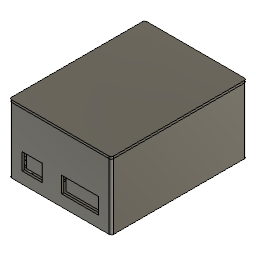
Case (Autodesk Fusion 360 design; units mm, degrees)
Autodesk Fusion 360 part; units mm, degrees
sketch "Base" plane through (0, 0, 0) normal (0, 0, 1) x (1, 0, 0) in component "PCB"
  line L0 (58.9, 60.9) -> (0, 60.9)
  line L1 (0, 60.9) -> (0, 0)
  line L2 (0, 0) -> (58.9, 0)
  line L3 (58.9, 0) -> (58.9, 60.9)
  circle A0 centre (3.45, 57.45) radius 1.6
  line L4 (29.45, 60.9) -> (29.45, 0) construction
  line L5 (0, 30.45) -> (58.9, 30.45) construction
  circle A1 centre (55.45, 57.45) radius 1.6
  circle A2 centre (3.45, 3.45) radius 1.6
  circle A3 centre (55.45, 3.45) radius 1.6
  dimension "d1" = 58.9
  dimension "d2" = 60.9
  dimension "d3" = 3.2
  dimension "d4" = 3.45
  dimension "d5" = 3.45
  constraint horizontal L0
  constraint vertical L1
  constraint horizontal L2
  constraint vertical L3
  constraint coincident L1.end L2.start
  constraint midpoint L0 L4.start
  constraint midpoint L2 L4.end
  constraint midpoint L1 L5.start
  constraint midpoint L3 L5.end
  constraint symmetric A0 L4 A1
  constraint symmetric A0 L5 A2
  constraint symmetric L5 A1 A3
  measures "d1" distance of L1.end L2.end
  measures "d2" distance of L0.end L1.end
  measures "d3" diameter of A0
  measures "d4" distance of L0 A0.centre
  measures "d5" distance of L1 A0.centre
extrude "Extrude1" add sketch "Base" along normal blind 24.2 makes body 1 in component "PCB"
sketch "USB port" plane through (0, 60.9, 0) normal (0, 1, 0) x (-1, 0, 0) in component "PCB"
  line L0 (-58.9, 0) -> (0, 0)
  line L1 (0, 0) -> (0, 24.2)
  line L2 (0, 24.2) -> (-58.9, 24.2)
  line L3 (-58.9, 24.2) -> (-58.9, 0)
  line L4 (-44.9, 16.5) -> (-36.9, 16.5)
  line L5 (-36.9, 16.5) -> (-36.9, 13.5)
  line L6 (-36.9, 13.5) -> (-44.9, 13.5)
  line L7 (-44.9, 13.5) -> (-44.9, 16.5)
  dimension "d8" = 8
  dimension "d9" = 3
  dimension "d10" = 14
  dimension "d11" = 13.5
  constraint horizontal L4
  constraint vertical L5
  constraint horizontal L6
  constraint vertical L7
  measures "d8" distance of L4.start L4.end
  measures "d9" distance of L4.start L6.end
  measures "d10" distance of L3 L7
  measures "d11" distance of L0 L6
extrude "Extrude2" add sketch "USB port" along normal blind 1 contours L4 L5 L6 L7 bodies 1 in component "PCB"
sketch "Base (2)" plane through (0, 0, 0) normal (0, 0, 1) x (1, 0, 0) in component "RJ45 breakout"
  line L0 (35.9, 21.4) -> (0, 21.4)
  line L1 (0, 21.4) -> (0, 0)
  line L2 (0, 0) -> (35.9, 0)
  line L3 (35.9, 0) -> (35.9, 21.4)
  circle A0 centre (4, 5) radius 1.6
  line L4 (17.95, 21.4) -> (17.95, 0) construction
  circle A1 centre (31.9, 5) radius 1.6
  dimension "d14" = 35.9
  dimension "d15" = 21.4
  dimension "d16" = 3.2
  dimension "d17" = 5
  dimension "d18" = 4
  constraint horizontal L0
  constraint vertical L1
  constraint horizontal L2
  constraint vertical L3
  constraint coincident L1.end L2.start
  constraint midpoint L0 L4.start
  constraint midpoint L2 L4.end
  constraint symmetric A0 L4 A1
  measures "d14" distance of L0.start L0.end
  measures "d15" distance of L0.end L1.end
  measures "d16" diameter of A0
  measures "d17" distance of L2 A0.centre
  measures "d18" distance of L1 A0.centre
extrude "Extrude1'" add sketch "Base (2)" along normal blind 1.5 separate body makes body 2 in component "RJ45 breakout"
sketch "Port" plane through (0, 0, 1.5) normal (0, 0, 1) x (-1, 0, 0) in component "RJ45 breakout"
  circle A0 centre (-31.9, -5) radius 1.6
  circle A1 centre (-4, -5) radius 1.6
  line L0 (-35.9, 0) -> (-35.9, -21.4)
  line L1 (-35.9, -21.4) -> (0, -21.4)
  line L2 (0, -21.4) -> (0, 0)
  line L3 (0, 0) -> (-35.9, 0)
  line L4 (-9.8, -13.3) -> (-26.1, -13.3)
  line L5 (-26.1, -13.3) -> (-26.1, 2.1)
  line L6 (-26.1, 2.1) -> (-9.8, 2.1)
  line L7 (-9.8, 2.1) -> (-9.8, -13.3)
  dimension "d21" = 16.3
  dimension "d22" = 15.4
  dimension "d23" = 2.1
  dimension "d24" = 35.9
  dimension "d25" = 9.8
  constraint horizontal L4
  constraint vertical L5
  constraint horizontal L6
  constraint vertical L7
  measures "d21" distance of L4.start L4.end
  measures "d22" distance of L4.start L6.end
  measures "d23" distance of L3 L6
  measures "d24" distance of L0.end L1.end
  measures "d25" distance of L2 L7
extrude "Extrude2'" add sketch "Port" along normal blind 13.3 contours L3 L5 L6 L7 | L3 L4 L5 L7 bodies 2 in component "RJ45 breakout"
sketch "Base (3)" plane through (0, 0, 0) normal (0, 0, 1) x (1, 0, 0) in component "UART to RS-232 converter"
  line L0 (31.6, 28) -> (0, 28)
  line L1 (0, 28) -> (0, 0)
  line L2 (0, 0) -> (31.6, 0)
  line L3 (31.6, 0) -> (31.6, 28)
  circle A0 centre (2.1, 25.7) radius 1.6
  line L4 (15.8, 28) -> (15.8, 0) construction
  circle A1 centre (29.5, 25.7) radius 1.6
  dimension "d28" = 28
  dimension "d29" = 31.6
  dimension "d30" = 3.2
  dimension "d31" = 2.1
  dimension "d32" = 2.3
  constraint horizontal L0
  constraint vertical L1
  constraint horizontal L2
  constraint vertical L3
  constraint coincident L1.end L2.start
  constraint midpoint L0 L4.start
  constraint midpoint L2 L4.end
  constraint symmetric A0 L4 A1
  measures "d28" distance of L0.end L1.end
  measures "d29" distance of L0.start L0.end
  measures "d30" diameter of A0
  measures "d31" distance of L1 A0.centre
  measures "d32" distance of L0 A0.centre
extrude "Extrude1''" add sketch "Base (3)" along normal blind 1.5 separate body makes body 3 in component "UART to RS-232 converter"
sketch "Port (2)" plane through (0, 0, 1.5) normal (0, 0, 1) x (-1, 0, 0) in component "UART to RS-232 converter"
  circle A0 centre (-29.5, -25.7) radius 1.6
  circle A1 centre (-2.1, -25.7) radius 1.6
  line L0 (-31.6, 0) -> (-31.6, -28)
  line L1 (-31.6, -28) -> (0, -28)
  line L2 (0, -28) -> (0, 0)
  line L3 (0, 0) -> (-31.6, 0)
  line L4 (0, -12.3) -> (-31.6, -12.3)
  line L5 (-31.6, -12.3) -> (-31.6, 17.9)
  line L6 (-31.6, 17.9) -> (0, 17.9)
  line L7 (0, 17.9) -> (0, -12.3)
  dimension "d35" = 30.2
  dimension "d36" = 12.3
  constraint horizontal L4
  constraint vertical L5
  constraint horizontal L6
  constraint vertical L7
  constraint collinear L2 L7
  constraint collinear L0 L5
  measures "d35" distance of L4.start L6.end
  measures "d36" distance of L3 L4
extrude "Extrude2''" add sketch "Port (2)" along normal blind 12.7 contours L0 L2 L3 L4 L5 L7 | L3 L5 L6 L7 bodies 3 in component "UART to RS-232 converter"
other "GeometricRelationship6"
sketch "Base (4)" plane through (0, 0, 0) normal (0, 0, 1) x (1, 0, 0) in component "Case"
  line L0 (-24.1768, 62.9) -> (65.1232, 62.9)
  line L1 (65.1232, 62.9) -> (65.1232, -56.9)
  line L2 (65.1232, -56.9) -> (-24.1768, -56.9)
  line L3 (-24.1768, -56.9) -> (-24.1768, 62.9)
  line L4 (-26.1768, 64.9) -> (67.1232, 64.9)
  line L5 (67.1232, 64.9) -> (67.1232, -58.9)
  line L6 (67.1232, -58.9) -> (-26.1768, -58.9)
  line L7 (-26.1768, -58.9) -> (-26.1768, 64.9)
  point P0 (-23.1768, -53.8)
  point P1 (54.3232, -55.9)
  point P2 (44.9, 61.9)
  point P3 (-13.3768, -55.9)
  dimension "d63" = 1
  dimension "d64" = 1
  dimension "d65" = 10.8
  dimension "d66" = 1
  dimension "d67" = 2
  dimension "d68" = 2
  dimension "d69" = 2
  dimension "d70" = 2
  dimension "d81" = 9.8
  constraint horizontal L0
  constraint vertical L1
  constraint horizontal L2
  constraint vertical L3
  constraint horizontal L4
  constraint vertical L5
  constraint horizontal L6
  constraint vertical L7
  measures "d63" distance of P0 L3
  measures "d64" distance of P1 L2
  measures "d65" distance of P1 L1
  measures "d66" distance of P2 L0
  measures "d67" distance of L0 L4
  measures "d68" distance of L3 L7
  measures "d69" distance of L1 L5
  measures "d70" distance of L2 L6
  measures "d81" horizontal distance of P0 P3
extrude "Extrude1'''" add sketch "Base (4)" along normal blind 10 separate body contours L0 L1 L2 L3 | L4 L5 L6 L7 makes body 4 in component "Case"
fillet "Fillet1" radius 2 4 edges at (67.1232, -58.9, 5) (67.1232, 64.9, 5) (-26.1768, 64.9, 5) (-26.1768, -58.9, 5) on bodies 4 in component "Case"
sketch "Walls" plane through (0, 0, 10) normal (0, 0, 1) x (-1, 0, 0) in component "Case"
  arc A0 (26.1768, 56.9) -> (24.1768, 58.9) centre (24.1768, 56.9) ccw
  line L0 (24.1768, 58.9) -> (-65.1232, 58.9)
  arc A1 (-65.1232, 58.9) -> (-67.1232, 56.9) centre (-65.1232, 56.9) ccw
  line L1 (-67.1232, 56.9) -> (-67.1232, -62.9)
  arc A2 (-67.1232, -62.9) -> (-65.1232, -64.9) centre (-65.1232, -62.9) ccw
  line L2 (-65.1232, -64.9) -> (24.1768, -64.9)
  arc A3 (24.1768, -64.9) -> (26.1768, -62.9) centre (24.1768, -62.9) ccw
  line L3 (26.1768, -62.9) -> (26.1768, 56.9)
  line L4 (24.1768, 56.9) -> (24.1768, -62.9)
  line L5 (-65.1232, 56.9) -> (24.1768, 56.9)
  line L6 (-65.1232, -62.9) -> (-65.1232, 56.9)
  line L7 (24.1768, -62.9) -> (-65.1232, -62.9)
extrude "Extrude2'''" add sketch "Walls" along normal blind 50 bodies 4 in component "Case"
other "GeometricRelationship8"
other "GeometricRelationship9"
sketch "Front port holes" plane through (0, -58.9, 0) normal (0, -1, 0) x (1, 0, 0) in component "Case"
  line L0 (-24.1768, 60) -> (-24.1768, 0)
  line L1 (-24.1768, 0) -> (65.1232, 0)
  line L2 (65.1232, 0) -> (65.1232, 60)
  line L3 (65.1232, 60) -> (-24.1768, 60)
  line L4 (-13.3768, 11.5) -> (2.9232, 11.5) construction
  line L5 (2.9232, 11.5) -> (2.9232, 24.8) construction
  line L6 (2.9232, 24.8) -> (-13.3768, 24.8) construction
  line L7 (-13.3768, 24.8) -> (-13.3768, 11.5) construction
  line L8 (22.7232, 11.5) -> (54.3232, 11.5) construction
  line L9 (54.3232, 11.5) -> (54.3232, 24.2) construction
  line L10 (54.3232, 24.2) -> (22.7232, 24.2) construction
  line L11 (22.7232, 24.2) -> (22.7232, 11.5) construction
  line L12 (-14.3768, 25.8) -> (3.9232, 25.8)
  line L13 (3.9232, 25.8) -> (3.9232, 10.5)
  line L14 (3.9232, 10.5) -> (-14.3768, 10.5)
  line L15 (-14.3768, 10.5) -> (-14.3768, 25.8)
  line L16 (21.7232, 25.2) -> (55.3232, 25.2)
  line L17 (55.3232, 25.2) -> (55.3232, 10.5)
  line L18 (55.3232, 10.5) -> (21.7232, 10.5)
  line L19 (21.7232, 10.5) -> (21.7232, 25.2)
  dimension "d82" = 1
  dimension "d83" = 1
  dimension "d84" = 1
  dimension "d85" = 1
  dimension "d86" = 1
  dimension "d87" = 1
  dimension "d88" = 1
  dimension "d89" = 1
  constraint horizontal L12
  constraint vertical L13
  constraint horizontal L14
  constraint vertical L15
  constraint horizontal L16
  constraint vertical L17
  constraint horizontal L18
  constraint vertical L19
  measures "d82" distance of L6 L12
  measures "d83" distance of L7 L15
  measures "d84" distance of L4 L14
  measures "d85" distance of L5 L13
  measures "d86" distance of L11 L19
  measures "d87" distance of L8 L18
  measures "d88" distance of L9 L17
  measures "d89" distance of L10 L16
extrude "Extrude3" cut sketch "Front port holes" against normal up to surface (2 mm away) contours L12 L13 L14 L15 | L16 L17 L18 L19 bodies 4 in component "Case"
sketch "Back port hole" plane through (0, 64.9, 0) normal (0, 1, 0) x (-1, 0, 0) in component "Case"
  line L0 (24.1768, 0) -> (24.1768, 60)
  line L1 (24.1768, 60) -> (-65.1232, 60)
  line L2 (-65.1232, 60) -> (-65.1232, 0)
  line L3 (-65.1232, 0) -> (24.1768, 0)
  line L4 (-35.9232, 23.5) -> (-27.9232, 23.5) construction
  line L5 (-27.9232, 23.5) -> (-27.9232, 26.5) construction
  line L6 (-27.9232, 26.5) -> (-35.9232, 26.5) construction
  line L7 (-35.9232, 26.5) -> (-35.9232, 23.5) construction
  line L8 (-37.9232, 29.5) -> (-25.9232, 29.5)
  line L9 (-25.9232, 29.5) -> (-25.9232, 20.5)
  line L10 (-25.9232, 20.5) -> (-37.9232, 20.5)
  line L11 (-37.9232, 20.5) -> (-37.9232, 29.5)
  dimension "d92" = 3
  dimension "d93" = 2
  dimension "d94" = 3
  dimension "d95" = 2
  constraint horizontal L8
  constraint vertical L9
  constraint horizontal L10
  constraint vertical L11
  measures "d92" distance of L6 L8
  measures "d93" distance of L7 L11
  measures "d94" distance of L4 L10
  measures "d95" distance of L5 L9
extrude "Extrude4" cut sketch "Back port hole" against normal up to surface (2 mm away) contours L8 L9 L10 L11 bodies 4 in component "Case"
sketch "Threaded insert holes" plane through (0, 0, 10) normal (0, 0, 1) x (-1, 0, 0) in component "Case"
  line L0 (24.1768, 56.9) -> (-65.1232, 56.9)
  line L1 (-65.1232, 56.9) -> (-65.1232, -62.9)
  line L2 (-65.1232, -62.9) -> (24.1768, -62.9)
  line L3 (24.1768, -62.9) -> (24.1768, 56.9)
  circle A0 centre (19.1768, 48.8) radius 1.6 construction
  circle A1 centre (-8.7232, 48.8) radius 1.6 construction
  circle A2 centre (-24.8232, 12.3) radius 1.6 construction
  circle A3 centre (-52.2232, 12.3) radius 1.6 construction
  circle A4 centre (-46.4732, -3.45) radius 1.6 construction
  circle A5 centre (5.5268, -3.45) radius 1.6 construction
  circle A6 centre (-46.4732, -57.45) radius 1.6 construction
  circle A7 centre (5.5268, -57.45) radius 1.6 construction
  circle A8 centre (5.5268, -57.45) radius 2
  circle A9 centre (-46.4732, -57.45) radius 2
  circle A10 centre (5.5268, -3.45) radius 2
  circle A11 centre (-46.4732, -3.45) radius 2
  circle A12 centre (-24.8232, 12.3) radius 2
  circle A13 centre (-52.2232, 12.3) radius 2
  circle A14 centre (19.1768, 48.8) radius 2
  circle A15 centre (-8.7232, 48.8) radius 2
  dimension "d98" = 4
  dimension "d99" = 4
  dimension "d100" = 4
  dimension "d101" = 4
  dimension "d102" = 4
  dimension "d103" = 4
  dimension "d104" = 4
  dimension "d105" = 4
  constraint coincident A7.centre A8.centre
  constraint coincident A6.centre A9.centre
  constraint coincident A5.centre A10.centre
  constraint coincident A4.centre A11.centre
  constraint coincident A2.centre A12.centre
  constraint coincident A3.centre A13.centre
  constraint coincident A0.centre A14.centre
  constraint coincident A1.centre A15.centre
  measures "d98" diameter of A8
  measures "d99" diameter of A9
  measures "d100" diameter of A10
  measures "d101" diameter of A11
  measures "d102" diameter of A12
  measures "d103" diameter of A13
  measures "d104" diameter of A14
  measures "d105" diameter of A15
extrude "Extrude5" cut sketch "Threaded insert holes" against normal blind 8 contours A8 | A9 | A10 | A11 | A12 | A13 | A14 | A15 bodies 4 in component "Case"
sketch "Lid 1" plane through (0, 0, 60) normal (0, 0, 1) x (-1, 0, 0) in component "Case"
  line L0 (24.1768, 56.9) -> (24.1768, -62.9)
  line L1 (24.1768, -62.9) -> (-65.1232, -62.9)
  line L2 (-65.1232, -62.9) -> (-65.1232, 56.9)
  line L3 (-65.1232, 56.9) -> (24.1768, 56.9)
  line L4 (26.1768, -62.9) -> (26.1768, 56.9)
  arc A0 (26.1768, 56.9) -> (24.1768, 58.9) centre (24.1768, 56.9) ccw
  line L5 (24.1768, 58.9) -> (-65.1232, 58.9)
  arc A1 (-65.1232, 58.9) -> (-67.1232, 56.9) centre (-65.1232, 56.9) ccw
  line L6 (-67.1232, 56.9) -> (-67.1232, -62.9)
  arc A2 (-67.1232, -62.9) -> (-65.1232, -64.9) centre (-65.1232, -62.9) ccw
  line L7 (-65.1232, -64.9) -> (24.1768, -64.9)
  arc A3 (24.1768, -64.9) -> (26.1768, -62.9) centre (24.1768, -62.9) ccw
  line L8 (23.6768, -62.4) -> (-64.6232, -62.4)
  line L9 (-64.6232, -62.4) -> (-64.6232, 56.4)
  line L10 (-64.6232, 56.4) -> (23.6768, 56.4)
  line L11 (23.6768, 56.4) -> (23.6768, -62.4)
  dimension "d108" = 0.5
  dimension "d109" = 0.5
  dimension "d110" = 0.5
  dimension "d111" = 0.5
  constraint horizontal L8
  constraint vertical L9
  constraint horizontal L10
  constraint vertical L11
  measures "d108" distance of L0 L11
  measures "d109" distance of L2 L9
  measures "d110" distance of L1 L8
  measures "d111" distance of L3 L10
extrude "Extrude6" add sketch "Lid 1" against normal blind 1 separate body contours L8 L9 L10 L11 makes body 5 in component "Case"
sketch "Lid 2" plane through (0, 0, 60) normal (0, 0, 1) x (-1, 0, 0) in component "Case"
  line L0 (23.6768, 56.4) -> (-64.6232, 56.4)
  line L1 (-64.6232, 56.4) -> (-64.6232, -62.4)
  line L2 (-64.6232, -62.4) -> (23.6768, -62.4)
  line L3 (23.6768, -62.4) -> (23.6768, 56.4)
  line L4 (-65.1232, -64.9) -> (24.1768, -64.9)
  arc A0 (24.1768, -64.9) -> (26.1768, -62.9) centre (24.1768, -62.9) ccw
  line L5 (26.1768, -62.9) -> (26.1768, 56.9)
  arc A1 (26.1768, 56.9) -> (24.1768, 58.9) centre (24.1768, 56.9) ccw
  line L6 (24.1768, 58.9) -> (-65.1232, 58.9)
  arc A2 (-65.1232, 58.9) -> (-67.1232, 56.9) centre (-65.1232, 56.9) ccw
  line L7 (-67.1232, 56.9) -> (-67.1232, -62.9)
  arc A3 (-67.1232, -62.9) -> (-65.1232, -64.9) centre (-65.1232, -62.9) ccw
extrude "Extrude7" add sketch "Lid 2" along normal blind 2 separate body contours L0 L1 L2 L3 | L4 A0 L5 A1 L6 A2 L7 A3 makes body 6 in component "Case"
combine "Combine1" operation add target body 5 tool bodies 6 in component "Case"
sketch "Sketch8" plane through (0, 0, 10) normal (0, 0, 1) x (-1, 0, 0) in component "Case"
  circle A0 centre (-52.2232, 12.3) radius 2
  circle A1 centre (-46.4732, -57.45) radius 2
  circle A2 centre (-46.4732, -3.45) radius 2
  circle A3 centre (-8.7232, 48.8) radius 2
  circle A4 centre (-24.8232, 12.3) radius 2
  circle A5 centre (5.5268, -57.45) radius 2
  circle A6 centre (5.5268, -3.45) radius 2
  circle A7 centre (19.1768, 48.8) radius 2
  line L0 (24.1768, 56.9) -> (-65.1232, 56.9)
  line L1 (-65.1232, 56.9) -> (-65.1232, -62.9)
  line L2 (-65.1232, -62.9) -> (24.1768, -62.9)
  line L3 (24.1768, -62.9) -> (24.1768, 56.9)
  circle A8 centre (5.5268, -57.45) radius 3.5
  circle A9 centre (5.5268, -57.45) radius 2 construction
  circle A10 centre (-46.4732, -57.45) radius 2 construction
  circle A11 centre (-46.4732, -3.45) radius 2 construction
  circle A12 centre (-52.2232, 12.3) radius 2 construction
  circle A13 centre (-24.8232, 12.3) radius 2 construction
  circle A14 centre (5.5268, -3.45) radius 2 construction
  circle A15 centre (19.1768, 48.8) radius 2 construction
  circle A16 centre (-8.7232, 48.8) radius 2 construction
  circle A17 centre (-46.4732, -57.45) radius 3.5
  circle A18 centre (-46.4732, -3.45) radius 3.5
  circle A19 centre (5.5268, -3.45) radius 3.5
  circle A20 centre (-24.8232, 12.3) radius 3.5
  circle A21 centre (-52.2232, 12.3) radius 3.5
  circle A22 centre (19.1768, 48.8) radius 3.5
  circle A23 centre (-8.7232, 48.8) radius 3.5
  dimension "d116" = 7
  dimension "d117" = 7
  dimension "d118" = 7
  dimension "d119" = 7
  dimension "d120" = 7
  dimension "d121" = 7
  dimension "d122" = 7
  dimension "d123" = 7
  constraint coincident A5.centre A8.centre
  constraint coincident A1.centre A10.centre
  constraint coincident A6.centre A14.centre
  constraint coincident A2.centre A11.centre
  constraint coincident A0.centre A12.centre
  constraint coincident A4.centre A13.centre
  constraint coincident A3.centre A16.centre
  constraint coincident A7.centre A15.centre
  measures "d116" diameter of A8
  measures "d117" diameter of A17
  measures "d118" diameter of A18
  measures "d119" diameter of A19
  measures "d120" diameter of A20
  measures "d121" diameter of A21
  measures "d122" diameter of A22
  measures "d123" diameter of A23
extrude "Extrude8" cut sketch "Sketch8" against normal up to surface (8 mm away) contours L0 L1 L2 L3 bodies 4 in component "Case"
component "PCB" placed x (1, 0, 0) y (0, 1, 0) z (0, 0, 1) at (-8.9768, 0, 10)
component "RJ45 breakout" placed x (1, 0, 0) y (0, 1, 0) z (0, 0, 1) at (-23.1768, -53.8, 10)
component "UART to RS-232 converter" placed x (1, 0, 0) y (0, 1, 0) z (0, 0, 1) at (22.7232, -38, 10)
component "Case" placed x (1, 0, 0) y (0, 1, 0) z (0, 0, 1) at (0, 0, 0)
equation "d4 = 1.85 mm + d3 / 2"
equation "d5 = d4"
equation "d17 = 3.4 mm + d16 / 2"
equation "d18 = 2.4 mm + d16 / 2"
equation "d25 = ( d24 - d21 ) / 2"
equation "d31 = 0.5 mm + d30 / 2"
equation "d32 = 0.7 mm + d30 / 2"
equation "d65 = d63 + d81"
equation "d67 = d70"
equation "d68 = d70"
equation "d69 = d70"
equation "d83 = d82"
equation "d84 = d82"
equation "d85 = d82"
equation "d86 = d82"
equation "d87 = d82"
equation "d88 = d82"
equation "d89 = d82"
equation "d94 = d92"
equation "d95 = d93"
equation "d109 = d108"
equation "d110 = d108"
equation "d111 = d108"
named bodies: "Body", "Lid"
